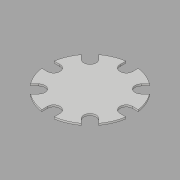
# Autodesk Inventor part: turntable
Saved by Autodesk Inventor 2017 (Build 210142000, 142)
## iProperties
Created: 2019-05-09
Part Number: turntable
Material: Generic
Document SubType Name: Modeling
Designer: Joe Sedutto
Density: 1 g/cm^3
Appearance: Default
Author: Joe Sedutto
Autodesk Inventor part; units mm, degrees
ref_plane "YZ Plane" through (0, 0, 0) normal (1, 0, 0) x (0, 1, 0)
ref_plane "XZ Plane" through (0, 0, 0) normal (0, 1, 0) x (-1, 0, 0)
ref_plane "XY Plane" through (0, 0, 0) normal (0, 0, 1) x (1, 0, 0)
sketch "Sketch1" plane through (0, 0, 0) normal (0, 1, 0) x (-1, 0, 0)
  circle A0 centre (0, 0) radius 34.925
  line L0 (0, 0) -> (0, -203.2) construction
  circle A1 centre (-143.6841, -59.5159) radius 34.925
  circle A2 centre (-203.2, -203.2) radius 34.925
  circle A3 centre (-143.6841, -346.8841) radius 34.925
  circle A4 centre (0, -406.4) radius 34.925
  circle A5 centre (143.6841, -346.8841) radius 34.925
  circle A6 centre (203.2, -203.2) radius 34.925
  circle A7 centre (143.6841, -59.5159) radius 34.925
  circle A8 centre (0, -203.2) radius 238.125
  dimension "d0" = 69.85
  dimension "d1" = 203.2
  dimension "d4" = 360
  constraints: 9 centre point, 2 coincident, 2 end point, 1 tangent, 1 vertical, 17 other
  measures "d0" diameter of A0
  measures "d1" distance of L0.end point (0, 0)
extrude "Extrusion1" add sketch "Sketch1" along normal blind 10
sketch "Sketch2" plane through (143.6841, 10, -59.5159) normal (0, 1, 0) x (1, 0, 0)
  arc A0 (-178.6091, -59.5159) -> (-108.7591, -59.5159) centre (-143.6841, -59.5159) ccw
  arc A1 (-178.6091, -91.8658) -> (-108.7591, -91.8658) centre (-143.6841, 143.6841) ccw
  line L0 (-108.7591, -59.5159) -> (-108.7591, -91.8658)
  line L1 (-178.6091, -59.5159) -> (-178.6091, -91.8658)
  circle A2 centre (-143.6841, -59.5159) radius 34.925 projected
  arc A3 (94.4409, 143.6841) -> (24.6957, 312.0639) centre (-143.6841, 143.6841) ccw projected
  arc A4 (-24.6957, -24.6957) -> (24.6957, 24.6957) centre (0, 0) ccw
  arc A5 (-1.8209, -47.5705) -> (47.5705, 1.8209) centre (-143.6841, 143.6841) ccw
  line L2 (24.6957, 24.6957) -> (47.5705, 1.8209)
  line L3 (-24.6957, -24.6957) -> (-1.8209, -47.5705)
  arc A6 (59.5159, 108.7591) -> (59.5159, 178.6091) centre (59.5159, 143.6841) ccw
  arc A7 (91.8658, 108.7591) -> (91.8658, 178.6091) centre (-143.6841, 143.6841) ccw
  line L4 (59.5159, 178.6091) -> (91.8658, 178.6091)
  line L5 (59.5159, 108.7591) -> (91.8658, 108.7591)
  arc A8 (24.6957, 262.6725) -> (-24.6957, 312.0639) centre (0, 287.3682) ccw
  arc A9 (47.5705, 285.5473) -> (-1.8209, 334.9387) centre (-143.6841, 143.6841) ccw
  line L6 (-24.6957, 312.0639) -> (-1.8209, 334.9387)
  line L7 (24.6957, 262.6725) -> (47.5705, 285.5473)
  arc A10 (-108.7591, 346.8841) -> (-178.6091, 346.8841) centre (-143.6841, 346.8841) ccw
  arc A11 (-108.7591, 379.234) -> (-178.6091, 379.234) centre (-143.6841, 143.6841) ccw
  line L8 (-178.6091, 346.8841) -> (-178.6091, 379.234)
  line L9 (-108.7591, 346.8841) -> (-108.7591, 379.234)
  arc A12 (-262.6725, 312.0639) -> (-312.0639, 262.6725) centre (-287.3682, 287.3682) ccw
  arc A13 (-285.5473, 334.9387) -> (-334.9387, 285.5473) centre (-143.6841, 143.6841) ccw
  line L10 (-312.0639, 262.6725) -> (-334.9387, 285.5473)
  line L11 (-262.6725, 312.0639) -> (-285.5473, 334.9387)
  arc A14 (-346.8841, 178.6091) -> (-346.8841, 108.7591) centre (-346.8841, 143.6841) ccw
  arc A15 (-379.234, 178.6091) -> (-379.234, 108.7591) centre (-143.6841, 143.6841) ccw
  line L12 (-346.8841, 108.7591) -> (-379.234, 108.7591)
  line L13 (-346.8841, 178.6091) -> (-379.234, 178.6091)
  arc A16 (-312.0639, 24.6957) -> (-262.6725, -24.6957) centre (-287.3682, 0) ccw
  arc A17 (-334.9387, 1.8209) -> (-285.5473, -47.5705) centre (-143.6841, 143.6841) ccw
  line L14 (-262.6725, -24.6957) -> (-285.5473, -47.5705)
  line L15 (-312.0639, 24.6957) -> (-334.9387, 1.8209)
  point P0 (-143.6841, -94.4409)
  point P1 (-143.6841, -94.4409)
  point P2 (24.6957, -24.6957)
  point P3 (24.6957, 312.0639)
  point P4 (-143.6841, 381.8091)
  point P5 (-312.0639, 312.0639)
  point P6 (-381.8091, 143.6841)
  point P7 (-312.0639, -24.6957)
  dimension "d10" = 360
  constraints: 42 point on circle, 32 end point, 16 centre point, 4 coincident, 2 tangent, 1 parallel, 1 vertical, 87 other
extrude "Extrusion2" cut sketch "Sketch2" against normal blind 10 contours A0 A1 L1 | A0 L0 A1 | A6 L4 A3 | A7 L5 A6 | L7 A8 A3 | A8 L6 A9 | A4 L2 A5 | A4 A5 L3 | A10 L8 A11 | A10 A11 L9 | A12 L10 A13 | A12 A13 L11 | A14 L12 A15 | A14 A15 L13 | A16 L14 A17 | A16 A17 L15
body "Solid1"
